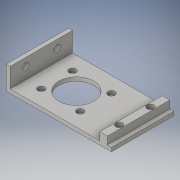
# Autodesk Inventor part: Upper Bracket of Elevator
Saved by Autodesk Inventor 2016 SP2 (Build 200236200, 236)
## iProperties
Created: 2018-01-27
Part Number: Upper Bracket of Elevator
Material: Generic
Document SubType Name: Modeling
Designer: CAD
Density: 1 g/cm^3
Appearance: Default
Author: CAD
Autodesk Inventor part; units mm, degrees
ref_plane "YZ Plane" through (0, 0, 0) normal (1, 0, 0) x (0, 1, 0)
ref_plane "XZ Plane" through (0, 0, 0) normal (0, 1, 0) x (-1, 0, 0)
ref_plane "XY Plane" through (0, 0, 0) normal (0, 0, 1) x (1, 0, 0)
sketch "Sketch1" plane through (0, 0, 0) normal (0, 0, 1) x (1, 0, 0)
  line L0 (0, 0) -> (85.725, 0)
  line L1 (0, 0) -> (0, 19.05)
  line L2 (85.725, 3.175) -> (3.175, 3.175)
  line L3 (3.175, 3.175) -> (3.175, 19.05)
  line L4 (0, 19.05) -> (3.175, 19.05)
  line L5 (85.725, 3.175) -> (85.725, 0)
  dimension "d0" = 85.725
  dimension "d1" = 19.05
  dimension "d2" = 3.175
  constraints: 12 end point, 2 horizontal, 1 perpendicular, 1 vertical, 1 other
  measures "d0" distance of L0.start L0.end
  measures "d1" distance of L0.start L1.end
  measures "d2" distance between parallel lines of L0 L2
extrude "Extrusion1" add sketch "Sketch1" along normal blind 50.8
sketch "Sketch2" plane through (3.175, 3.175, 0) normal (0, 1, 0) x (1, 0, 0)
  line L0 (82.55, 0) -> (0, 0) projected
  line L1 (82.55, -50.8) -> (0, -50.8) projected
  line L2 (82.55, 0) -> (82.55, -50.8) projected
  point P0 (-3.175, 0)
  point P1 (12.7, -38.1)
  point P2 (12.7, -12.7)
  point P3 (44.45, -38.1)
  point P4 (44.45, -12.7)
  point P5 (76.2, -38.1)
  point P6 (76.2, -12.7)
  dimension "d5" = 12.7
  dimension "d6" = 12.7
  dimension "d7" = 12.7
  dimension "d8" = 12.7
  dimension "d9" = 12.7
  dimension "d10" = 12.7
  dimension "d11" = 6.35
  dimension "d12" = 6.35
  dimension "d13" = 38.1
  dimension "d14" = 38.1
  dimension "d15" = 31.75
  dimension "d16" = 31.75
  measures "d5" distance from line of L0 point (76.2, -12.7)
  measures "d6" distance from line of L0 point (44.45, -12.7)
  measures "d7" distance from line of L0 point (12.7, -12.7)
  measures "d8" distance from line of L1 point (12.7, -38.1)
  measures "d9" distance from line of L1 point (44.45, -38.1)
  measures "d10" distance from line of L1 point (76.2, -38.1)
  measures "d11" distance from line of L2 point (76.2, -38.1)
  measures "d12" distance from line of L2 point (76.2, -12.7)
  measures "d13" distance from line of L2 point (44.45, -12.7)
  measures "d14" distance from line of L2 point (44.45, -38.1)
  measures "d15" distance of point (44.45, -38.1) point (12.7, -38.1)
  measures "d16" distance of point (44.45, -12.7) point (12.7, -12.7)
hole "Hole1" at (15.875, 3.175, 38.1) at (15.875, 3.175, 12.7) at (47.625, 3.175, 38.1) at (47.625, 3.175, 12.7) at (79.375, 3.175, 38.1) at (79.375, 3.175, 12.7) direction (0, -1, 0) diameter 5.5563 end through all
sketch "Sketch3" plane through (3.175, 3.175, 0) normal (1, 0, 0) x (0, 0, -1)
  line L0 (0, 0) -> (0, 15.875) projected
  line L1 (-50.8, 0) -> (-50.8, 15.875) projected
  line L2 (0, 0) -> (-50.8, 0) projected
  point P0 (0, -3.175)
  point P1 (-38.1, 9.525)
  point P2 (-12.7, 9.525)
  dimension "d24" = 12.7
  dimension "d25" = 12.7
  dimension "d26" = 9.525
  dimension "d27" = 9.525
  measures "d24" distance from line of L0 point (-12.7, 9.525)
  measures "d25" distance from line of L1 point (-38.1, 9.525)
  measures "d26" distance from line of L2 point (-38.1, 9.525)
  measures "d27" distance from line of L2 point (-12.7, 9.525)
hole "Hole2" at (3.175, 12.7, 38.1) at (3.175, 12.7, 12.7) direction (-1, 0, 0) diameter 5.5563 end through all
sketch "Sketch4" plane through (0, 0, 0) normal (0, -1, 0) x (1, 0, 0)
  line L0 (85.725, 50.8) -> (3.175, 50.8) projected
  line L1 (76.327, 50.8) -> (76.327, 0)
  line L2 (85.725, 0) -> (3.175, 0) projected
  line L3 (82.423, 50.8) -> (82.423, 0)
  line L4 (76.327, 0) -> (82.423, 0)
  line L5 (76.327, 50.8) -> (82.423, 50.8)
  circle A0 centre (79.375, 38.1) radius 2.7781 projected
  circle A1 centre (79.375, 12.7) radius 2.7781 projected
  point P0 (0, 0)
  dimension "d35" = 3.048
  dimension "d36" = 3.048
  constraints: 8 end point, 4 point on line, 2 collinear, 1 parallel, 1 vertical
  measures "d35" distance from line of L1 A1.centre
  measures "d36" distance from line of L3 A0.centre
extrude "Extrusion2" add sketch "Sketch4" against normal blind 9.525
sketch "Sketch5" plane through (0, 0, 0) normal (0, -1, 0) x (1, 0, 0)
  circle A0 centre (47.625, 38.1) radius 2.7781 projected
  circle A1 centre (15.875, 12.7) radius 2.7781 projected
  point P0 (0, 0)
  point P1 (31.75, 25.4)
  dimension "d41" = 15.875
  dimension "d42" = 12.7
  measures "d41" horizontal distance of A1.centre point (31.75, 25.4)
  measures "d42" vertical distance of A0.centre point (31.75, 25.4)
hole "Hole3" at (31.75, 0, 25.4) direction (0, 1, 0) diameter 28.575 end through all
body "Solid1"
